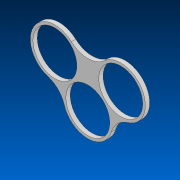
# Autodesk Inventor part: Flywheel Gearbox Holder
Saved by Autodesk Inventor 2022 (Build 260153000, 153)
## iProperties
Created: 2022-04-22
Part Number: Flywheel Gearbox Holder
Material: Generic
Document SubType Name: Modeling
Designer: score_nygvs6w
Density: 1 g/cm^3
Appearance: Default
Author: score_nygvs6w
Autodesk Inventor part; units mm, degrees
ref_plane "YZ Plane" through (0, 0, 0) normal (1, 0, 0) x (0, 1, 0)
ref_plane "XZ Plane" through (0, 0, 0) normal (0, 1, 0) x (-1, 0, 0)
ref_plane "XY Plane" through (0, 0, 0) normal (0, 0, 1) x (1, 0, 0)
sketch "Sketch1" plane through (0, 0, 0) normal (0, 0, 1) x (1, 0, 0)
  circle A0 centre (0, 0) radius 32.385
  circle A1 centre (-48.4934, 48.4934) radius 32.385
  circle A2 centre (48.4934, 48.4934) radius 32.385
  circle A3 centre (0, 0) radius 68.58 construction
  line L0 (-48.4934, 48.4934) -> (48.4934, 48.4934) construction
  circle A4 centre (-48.4934, -48.4934) radius 32.385 construction
  circle A5 centre (48.4934, -48.4934) radius 32.385 construction
  line L1 (-48.4934, 48.4934) -> (-48.4934, -48.4934) construction
  circle A6 centre (0, 0) radius 36.195
  circle A7 centre (-48.4934, 48.4934) radius 36.195
  circle A8 centre (48.4934, 48.4934) radius 36.195
  arc A9 (-24.2467, 75.3667) -> (24.2467, 75.3667) centre (0, 102.24) ccw
  arc A10 (-34.6636, -10.4169) -> (-58.9103, 13.8298) centre (-69.3272, -20.8338) ccw
  arc A11 (58.9103, 13.8298) -> (34.6636, -10.4169) centre (69.3272, -20.8338) ccw
  dimension "d0" = 137.16
  dimension "d1" = 64.77
  constraints: 16 point on circle, 12 centre point, 9 tangent, 7 equal radius, 4 end point, 2 coincident, 2 horizontal alignment, 2 vertical alignment, 1 horizontal, 1 perpendicular, 1 vertical
  measures "d0" diameter of A3
  measures "d1" diameter of A0
extrude "Extrusion1" add sketch "Sketch1" along normal blind 6.35 contours A0 A8 A6 A7 | A0 A7 A6 A8 | A8 A6 | A7 A6 | A8 A6 | A6 A7 A9 A8 | A8 A11 A6 | A7 A6 | A6 A10 A7
body "Solid1"
